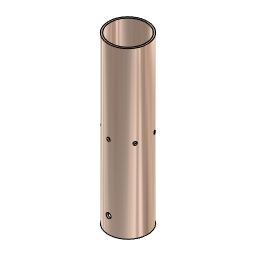
SHVFeedthroughFilter (Autodesk Fusion 360 archive; units mm, degrees)
design "OuterTube"
Autodesk Fusion 360 part; units mm, degrees
sketch "Sketch1" plane through (0, 0, 0) normal (0, 0, 1) x (1, 0, 0)
  circle A0 centre (0, 0) radius 9.525
  circle A1 centre (0, 0) radius 8.7122
  dimension "d1" = 19.05
  dimension "d2" = 0.8128
  constraint coincident A0.centre A1.centre
  constraint concentric A0 A1
  measures "d1" diameter of A0
  measures "d2" distance of A0 A1
extrude "Extrude1" add sketch "Sketch1" along normal blind 80.35
sketch "Sketch2" plane through (0, 0, 0) normal (0, 1, 0) x (1, 0, 0)
  point P0 (0, -8)
  dimension "d8" = 8
  measures "d8" distance of origin P0
hole "Hole1" at (0, 0, 8) direction (0, -1, 0) diameter 2.3813 depth 30 tip angle 118
sketch "Sketch3" plane through (0, 0, 0) normal (0, 1, 0) x (1, 0, 0)
  point P0 (0, -40.175)
  dimension "d9" = 40.175
  measures "d9" distance of origin P0
hole "Hole2" at (0, 0, 40.175) direction (0, -1, 0) diameter 1.5875 depth 20 tip angle 118
pattern_circular "C-Pattern1" count 6 over 360 about axis through (0, 0, 1.75) along (0, 0, 1) of "Hole2"
equation "d3 = 74 mm + 0.25 in"
equation "d6 = 3 in / 32"
equation "d9 = 37 mm + 0.125 in"
equation "d11 = 1 in / 16"

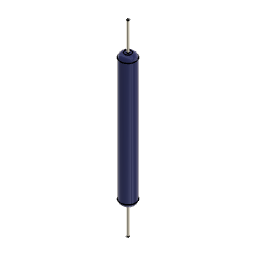
design "MOX1125-22"
Autodesk Fusion 360 part; units mm, degrees
sketch "Sketch1" plane through (0, 0, 0) normal (0, 0, 1) x (1, 0, 0)
  circle A0 centre (0, 0) radius 1.78
  dimension "d1" = 3.56
  constraint coincident A0.centre origin
  measures "d1" diameter of A0
extrude "Extrude1" add sketch "Sketch1" along normal mid plane 30.73 makes body 1
sketch "Sketch2" plane through (0, 0, 15.365) normal (0, 0, 1) x (-1, 0, 0)
  circle A0 centre (0, 0) radius 1.78
  circle A1 centre (0, 0) radius 0.254
  dimension "d4" = 0.508
  constraint concentric A0 A1
  measures "d4" diameter of A1
extrude "Extrude2" add sketch "Sketch2" along normal blind 6.63 separate body contours A1 makes body 2
mirror "Mirror1" about plane through (0, 0, 0) normal (0, 0, 1) of "Extrude2" makes body 3
fillet "Fillet1" radius 1 2 edges at (-1.6595, -0.6437, 15.365) (-1.6595, 0.6437, -15.365) on bodies 1
equation "d2 = 30.73 mm / 2"

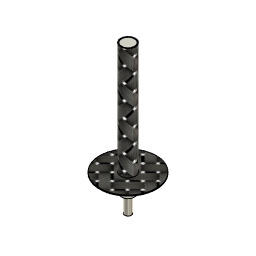
design "Cable"
Autodesk Fusion 360 part; units mm, degrees
sketch "Sketch1" plane through (0, 0, 0) normal (0, 0, 1) x (1, 0, 0)
  circle A0 centre (0, 0) radius 1.5
  dimension "d1" = 3
  constraint coincident A0.centre origin
  measures "d1" diameter of A0
extrude "Extrude1" add sketch "Sketch1" along normal blind 30 makes body 1
sketch "Sketch2" plane through (0, 0, 30) normal (0, 0, 1) x (-1, 0, 0)
  circle A0 centre (0, 0) radius 1.5
  circle A1 centre (0, 0) radius 1.7
  dimension "d4" = 0.2
extrude "Extrude2" add sketch "Sketch2" against normal blind 25.753 separate body makes body 2
sketch "Sketch3" plane through (0, 0, 4.247) normal (0, 0, -1) x (1, 0, 0)
  circle A0 centre (0, 0) radius 1.5
  circle A1 centre (0, 0) radius 1.7
  circle A2 centre (0, 0) radius 6.5
  dimension "d7" = 13
  constraint concentric A0 A2
  measures "d7" diameter of A2
extrude "Extrude3" add sketch "Sketch3" along normal blind 0.2 separate body contours A1 | A2 makes body 3
sketch "Sketch4" plane through (0, 0, 0) normal (0, 0, -1) x (1, 0, 0)
  circle A0 centre (0, 0) radius 1.5
  circle A1 centre (0, 0) radius 0.75
  dimension "d10" = 1.5
  constraint coincident A0.centre A1.centre
  measures "d10" diameter of A1
extrude "Extrude4" add sketch "Sketch4" along normal blind 4.0005 separate body contours A1 makes body 4
combine "Combine1" operation add target body 3 tool bodies 2
equation "d11 = 0.315 in / 2"

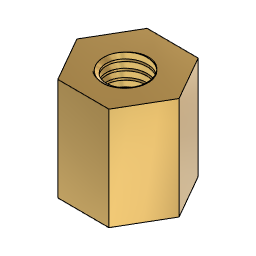
design "CapacitorArrayCenter"
Autodesk Fusion 360 part; units mm, degrees
sketch "Sketch1" plane through (0, 0, 0) normal (0, 0, 1) x (1, 0, 0)
  line L0 (1.5999, 2.7429) -> (-1.5755, 2.757)
  line L1 (-1.5755, 2.757) -> (-3.1754, 0.0141)
  line L2 (-3.1754, 0.0141) -> (-1.5999, -2.7429)
  line L3 (-1.5999, -2.7429) -> (1.5755, -2.757)
  line L4 (1.5755, -2.757) -> (3.1754, -0.0141)
  line L5 (3.1754, -0.0141) -> (1.5999, 2.7429)
  dimension "d1" = 5.5
  measures "d1" distance of L0 L3
extrude "Extrude1" add sketch "Sketch1" along normal mid plane 6.35
sketch "Sketch2" plane through (0, 0, 3.175) normal (0, 0, 1) x (-1, 0, 0)
  line L0 (-3.1754, 0.0141) -> (-1.5999, -2.7429)
  line L1 (-1.5999, -2.7429) -> (1.5755, -2.757)
  line L2 (1.5755, -2.757) -> (3.1754, -0.0141)
  line L3 (3.1754, -0.0141) -> (1.5999, 2.7429)
  line L4 (1.5999, 2.7429) -> (-1.5755, 2.757)
  line L5 (-1.5755, 2.757) -> (-3.1754, 0.0141)
hole "Hole1" at (0, 0, 3.175) direction (0, 0, -1) diameter 2.529 end through all
thread "Thread1" "ISO Metric profile 3.0 M3x0.5 6H" major diameter 3.086 minor diameter 2.529 pitch 0.5 angle 60 modelled right hand crest width 0.1368 on face at (0.1259, -1.2582, 1.0583) crest through (1.2645, 0, 3.05)

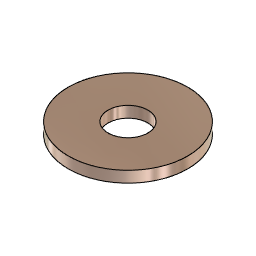
design "Washer"
Autodesk Fusion 360 part; units mm, degrees
sketch "Sketch1" plane through (0, 0, 0) normal (0, 0, 1) x (1, 0, 0)
  circle A0 centre (0, 0) radius 9.525
  circle A1 centre (0, 0) radius 3.175
  dimension "d1" = 19.05
  dimension "d2" = 6.35
  constraint coincident A0.centre A1.centre
  measures "d1" diameter of A0
  measures "d2" diameter of A1
extrude "Extrude1" add sketch "Sketch1" along normal blind 1.778

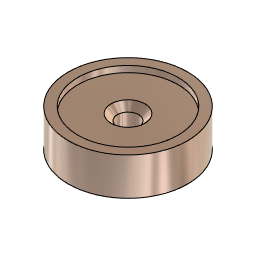
design "Grommet"
Autodesk Fusion 360 part; units mm, degrees
sketch "Sketch1" plane through (0, 0, 0) normal (0, 1, 0) x (1, 0, 0)
  line L0 (8, 0) -> (8, 1)
  line L1 (8, 0) -> (9.525, 0)
  line L2 (9.525, 0) -> (9.525, 6)
  line L3 (9.525, 6) -> (1.7, 6)
  line L4 (1.7, 6) -> (1.7, 1)
  line L5 (1.7, 1) -> (8, 1)
  dimension "d1" = 9.525
  dimension "d2" = 1.7
  dimension "d3" = 1
  dimension "d4" = 5
  dimension "d5" = 8
  constraint perpendicular L0 L1
  constraint perpendicular L1 L2
  constraint perpendicular L2 L3
  constraint perpendicular L3 L4
  constraint perpendicular L0 L5
  constraint horizontal L1
  constraint horizontal origin L0.start
  measures "d1" distance of origin L2
  measures "d2" distance of origin L4
  measures "d3" distance of L0.start L0.end
  measures "d4" distance of L3.end L4.end
  measures "d5" distance of origin L0.start
revolve "Revolve2" add sketch "Sketch1" angle 360 about axis through (0, 0, 1.75) along (0, 0, 1)
chamfer "Chamfer1" distance 1 angle 45 1 edges at (-1.585, -0.6147, -1)
equation "d1 = 0.75 in / 2"
